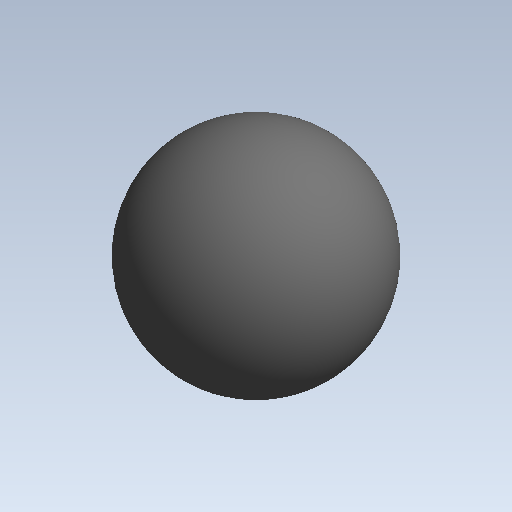
# Autodesk Inventor part: MF126ZZ Ball
Saved by Autodesk Inventor 2020.2 (Build 242310000, 310)
## iProperties
Part Number: MF126ZZ Ball
Material: 一般
Catalog Web Link: www.cadenas.de
Description: shielded_type_zz_zzs_B-
Vendor: NSK_RB
Document SubType Name: Modeling
Designer: partserver
Manufacturer: NSK_RB
Mass: 0.00305363 g
Surface Area: 0.101788 cm^2
Volume: 0.00305363 cm^3
Density: 1 g/cm^3
Appearance: PSOLRGB-128-128-128
Category: PARTsolutions
Company: NSK_RB
PSOL_IDENT_0: {$CADENAS_DATA\23d-libs\nsk_rb\roller_bearings\deep_groove_bb\exstra_small_miniatur_bb\metric_design
PSOL_IDENT_1: _with_flange\shielded_type_zz_zzs_b_1.prj},181 {VTYP=3D},{NB=MF126ZZ Ball},{LINA=MF126ZZ Ball},{NN=s
PSOL_IDENT_2: hielded_type_zz_zzs_B},{DATE=10.04.2020 04:57:39},{GEOMDATE=04.01.2008 00:00:00},{VERSION=},{LINEID=
PSOL_IDENT_3: 570},{WBVAR=},{WBNUMERIC=}  {NB=MF126ZZ Ball},{LINA=MF126ZZ Ball},{KT=DUMMY},{IDNR=},{STAN=},{ORDER=
PSOL_IDENT_4: MF126ZZ},{SD=6.0},{X=6.0},{D=12},{DD=12},{DD1=0.0},{D2=13.6},{DD2=13.6},{B=0.0},{B1=4.0},{CC1=0.0},{
PSOL_IDENT_5: C2=0.8},{CC2=0.8},{R=0.00},{R1=0.15},{DI1=7.73},{DI2=7.20},{SDE1=10.19},{SDE2=10.90},{CR1=715},{COR1=
PSOL_IDENT_6: 292},{CR2=73},{COR2=30.0},{LG=43000},{LO=50000},{DA=0.0},{DB=7.2},{RA=0.00},{RB=0.15},{MASS=1.94},{S
PSOL_IDENT_7: C=1}
NB: MF126ZZ Ball
NN: shielded_type_zz_zzs_B
NBSYN: $ORDER. Ball
LINA: MF126ZZ Ball
CATALOG: NSK Rolling Bearing
ORDER: MF126ZZ
SD: 6
X: 6
D: 12
DD: 12
DD1: 0
D2: 13.6
DD2: 13.6
B: 0
B1: 4
CC1: 0
C2: 0.8
CC2: 0.8
R: 0
R1: 0.15
DI1: 7.73
DI2: 7.2
SDE1: 10.19
SDE2: 10.9
CR1: 715
COR1: 292
CR2: 73
COR2: 30
LG: 43000
LO: 50000
DA: 0
DB: 7.2
RA: 0
RB: 0.15
MASS: 1.94
SC: 1
SUPPLIER: NSK_RB
ARTICLENO: MF126ZZ Ball
BOMINFO: MF126ZZ Ball
CREATOR: CADENAS GmbH
Title: MF126ZZ Ball
Author: Cadenas PARTsolutions
Autodesk Inventor part; units mm, degrees
sketch "Sketch_1" plane through (0, 0, 0) normal (0, 0, 1) x (1, 0, 0)
  line L0 (0.9, 0) -> (-0.9, 0)
  arc A0 (0.9, 0) -> (-0.9, 0) centre (0, 0) ccw
  line L1 (0.9, 0) -> (-0.9, 0)
  constraints: 4 end point, 2 point on circle, 1 centre point
revolve "Revolution1" add sketch "Sketch_1" angle 360 about axis through (0.9, 0, 0) along (1, 0, 0)
ref_plane "ip_st_1_XY" through (0, 0, 0) normal (-1, 0, 0) x (0, 0, -1)
ref_plane "ip_st_1_YZ" through (0, 0, 0) normal (0, 0, -1) x (0, -1, 0)
ref_plane "ip_st_1_ZX" through (0, 0, 0) normal (0, -1, 0) x (-1, 0, 0)
body "Solid1"
